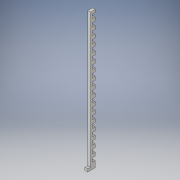
# Autodesk Inventor part: 000.208 - Заглушка
Saved by Autodesk Inventor 2019 (Build 230136000, 136)
## iProperties
Created: 2020-04-11
Part Number: 000.208 - Заглушка
Material: Типовые
Document SubType Name: Modeling
Designer: Петров Иван
Density: 1 g/cm^3
Appearance: По умолчанию
Author: Петров Иван
Autodesk Inventor part; units mm, degrees
ref_plane "YZ Plane" through (0, 0, 0) normal (1, 0, 0) x (0, 1, 0)
ref_plane "XZ Plane" through (0, 0, 0) normal (0, 1, 0) x (-1, 0, 0)
ref_plane "XY Plane" through (0, 0, 0) normal (0, 0, 1) x (1, 0, 0)
sketch "Эскиз1" plane through (0, 0, 0) normal (1, 0, 0) x (0, 1, 0)
  line L0 (-75, -22.5) -> (-75, -35.5)
  line L1 (75, -30.5) -> (75, -25.5)
  line L2 (75, -25.5) -> (-75, -25.5)
  line L3 (-75, -25.5) -> (-75, -35.5)
  line L4 (-72, -22.5) -> (-72, -35.5)
  line L5 (-72, -22.5) -> (-72, -35.5)
  line L6 (-68, -35.5) -> (-72, -35.5)
  line L7 (-68, -32.5) -> (-68, -35.5)
  line L8 (-68, -32.5) -> (-64, -32.5)
  line L9 (-64, -35.5) -> (-64, -32.5)
  line L10 (-60, -35.5) -> (-64, -35.5)
  line L11 (-60, -32.5) -> (-60, -35.5)
  line L12 (-60, -32.5) -> (-56, -32.5)
  line L13 (-56, -35.5) -> (-56, -32.5)
  line L14 (-52, -35.5) -> (-56, -35.5)
  line L15 (-52, -32.5) -> (-52, -35.5)
  line L16 (-52, -32.5) -> (-48, -32.5)
  line L17 (-48, -35.5) -> (-48, -32.5)
  line L18 (-44, -35.5) -> (-48, -35.5)
  line L19 (-44, -32.5) -> (-44, -35.5)
  line L20 (-44, -32.5) -> (-40, -32.5)
  line L21 (-40, -35.5) -> (-40, -32.5)
  line L22 (-36, -35.5) -> (-40, -35.5)
  line L23 (-36, -32.5) -> (-36, -35.5)
  line L24 (-36, -32.5) -> (-32, -32.5)
  line L25 (-32, -35.5) -> (-32, -32.5)
  line L26 (-28, -35.5) -> (-32, -35.5)
  line L27 (-28, -32.5) -> (-28, -35.5)
  line L28 (-28, -32.5) -> (-24, -32.5)
  line L29 (-24, -35.5) -> (-24, -32.5)
  line L30 (-20, -35.5) -> (-24, -35.5)
  line L31 (-20, -32.5) -> (-20, -35.5)
  line L32 (-20, -32.5) -> (-16, -32.5)
  line L33 (-16, -35.5) -> (-16, -32.5)
  line L34 (-12, -35.5) -> (-16, -35.5)
  line L35 (-12, -32.5) -> (-12, -35.5)
  line L36 (-12, -32.5) -> (-8, -32.5)
  line L37 (-8, -35.5) -> (-8, -32.5)
  line L38 (-4, -35.5) -> (-8, -35.5)
  line L39 (-4, -32.5) -> (-4, -35.5)
  line L40 (-4, -32.5) -> (0, -32.5)
  line L41 (0, -35.5) -> (0, -32.5)
  line L42 (4, -35.5) -> (0, -35.5)
  line L43 (4, -32.5) -> (4, -35.5)
  line L44 (4, -32.5) -> (8, -32.5)
  line L45 (8, -35.5) -> (8, -32.5)
  line L46 (12, -35.5) -> (8, -35.5)
  line L47 (12, -32.5) -> (12, -35.5)
  line L48 (12, -32.5) -> (16, -32.5)
  line L49 (16, -35.5) -> (16, -32.5)
  line L50 (20, -35.5) -> (16, -35.5)
  line L51 (20, -32.5) -> (20, -35.5)
  line L52 (20, -32.5) -> (24, -32.5)
  line L53 (24, -35.5) -> (24, -32.5)
  line L54 (28, -35.5) -> (24, -35.5)
  line L55 (28, -32.5) -> (28, -35.5)
  line L56 (28, -32.5) -> (32, -32.5)
  line L57 (32, -35.5) -> (32, -32.5)
  line L58 (36, -35.5) -> (32, -35.5)
  line L59 (36, -32.5) -> (36, -35.5)
  line L60 (36, -32.5) -> (40, -32.5)
  line L61 (40, -35.5) -> (40, -32.5)
  line L62 (44, -35.5) -> (40, -35.5)
  line L63 (44, -32.5) -> (44, -35.5)
  line L64 (44, -32.5) -> (48, -32.5)
  line L65 (48, -35.5) -> (48, -32.5)
  line L66 (52, -35.5) -> (48, -35.5)
  line L67 (52, -32.5) -> (52, -35.5)
  line L68 (52, -32.5) -> (56, -32.5)
  line L69 (56, -35.5) -> (56, -32.5)
  line L70 (60, -35.5) -> (56, -35.5)
  line L71 (60, -32.5) -> (60, -35.5)
  line L72 (60, -32.5) -> (64, -32.5)
  line L73 (64, -35.5) -> (64, -32.5)
  line L74 (68, -35.5) -> (64, -35.5)
  line L75 (68, -32.5) -> (68, -35.5)
  line L76 (68, -32.5) -> (72, -32.5)
  line L77 (72, -32.5) -> (72, -27.5)
  line L78 (72, -27.5) -> (75, -27.5)
  line L79 (75, -27.5) -> (75, -22.5)
  line L80 (-75, -35.5) -> (-68, -35.5)
  line L81 (-64, -35.5) -> (-60, -35.5)
  line L82 (-56, -35.5) -> (-52, -35.5)
  line L83 (-48, -35.5) -> (-44, -35.5)
  line L84 (-40, -35.5) -> (-36, -35.5)
  line L85 (-32, -35.5) -> (-28, -35.5)
  line L86 (-24, -35.5) -> (-20, -35.5)
  line L87 (-16, -35.5) -> (-12, -35.5)
  line L88 (-8, -35.5) -> (-4, -35.5)
  line L89 (0, -35.5) -> (4, -35.5)
  line L90 (8, -35.5) -> (12, -35.5)
  line L91 (16, -35.5) -> (20, -35.5)
  line L92 (24, -35.5) -> (28, -35.5)
  line L93 (32, -35.5) -> (36, -35.5)
  line L94 (40, -35.5) -> (44, -35.5)
  line L95 (48, -35.5) -> (52, -35.5)
  line L96 (56, -35.5) -> (60, -35.5)
  line L97 (64, -35.5) -> (68, -35.5)
  line L98 (-75, -25.5) -> (-72, -25.5)
  line L99 (-72, -25.5) -> (-72, -27.5)
  line L100 (-72, -27.5) -> (-75, -27.5)
  line L101 (-75, -27.5) -> (-75, -25.5)
  dimension "d0" = 5
  dimension "d3" = 2
  constraints: 204 end point, 21 parallel, 19 horizontal, 19 perpendicular, 2 point on line, 1 vertical
  measures "d0" distance of L1.end L1.start
  measures "d3" distance of L98.end L99.end
extrude "Выдавливание1" add sketch "Эскиз1" along normal blind 3 contours L100 L4 L80 L0 | L2 L1 L78 L77 L76 L75 L74 L73 L72 L71 L70 L69 L68 L67 L66 L65 L64 L63 L62 L61 L60 L59 L58 L57 L56 L55 L54 L53 L52 L51 L50 L49 L48 L47 L46 L45 L44 L43 L42 L41 L40 L39 L38 L37 L36 L35 L34 L33 L32 L31 L30 L29 L28 L27 L26 L25 L24 L23 L22 L21 L20 L19 L18 L17 L16 L15 L14 L13 L12 L11 L10 L9 L8 L7 L6 L4
sketch "Эскиз2" plane through (3, 0, 0) normal (1, 0, 0) x (0, 0, -1)
  line L0 (27.5, 72) -> (27.5, 75) projected
  line L1 (27.5, 75) -> (35.5, 75)
  line L2 (35.5, 75) -> (35.5, 72)
  line L3 (35.5, 72) -> (27.5, 72)
  line L4 (27.5, 72) -> (27.5, 75)
  point P0 (0, 0)
  dimension "d4" = 3
  constraints: 8 end point, 2 parallel, 1 horizontal, 1 perpendicular
  measures "d4" distance of L1.end L2.end
extrude "Выдавливание2" add sketch "Эскиз2" against normal blind 3
move faces "Перенос1" translate (0, 0, -5) faces at (1, 26, -25.5)
